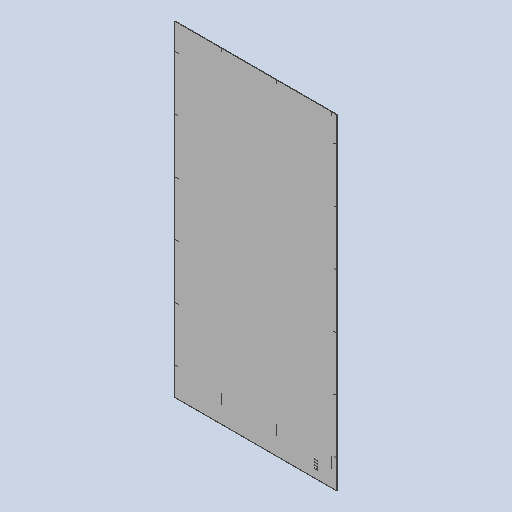
# Autodesk Inventor part: GBK 2221 shield 5
Saved by Autodesk Inventor 2026 (Build 300175000, 175)
## iProperties
Created: 2026-04-17
Part Number: GBK 2221 shield 5
Material: Steel
Document SubType Name: Sheet Metal
Designer: pokla
Stock Number: 2225
Mass: 138487 g
Surface Area: 88564.8 cm^2
Volume: 17641.6 cm^3
Density: 7.85 g/cm^3
Flat Pattern Width: 148 cm
Flat Pattern Length: 298 cm
Flat Pattern Area: 44104 cm^2
Sheet Metal Rule: По умолчанию_мм
Sheet Metal Width: 1480,000 мм
Sheet Metal Length: 2980,000 мм
Sheet Metal Area: 4410400,000 мм^2
Appearance: Default
Author: admin
Autodesk Inventor part; units mm, degrees
ref_plane "YZ Plane" through (0, 0, 0) normal (1, 0, 0) x (0, 1, 0)
ref_plane "XZ Plane" through (0, 0, 0) normal (0, 1, 0) x (-1, 0, 0)
ref_plane "XY Plane" through (0, 0, 0) normal (0, 0, 1) x (1, 0, 0)
sketch "Sketch1" plane through (0, 0, 0) normal (0, 0, 1) x (1, 0, 0)
  line L0 (740, -1490) -> (-740, -1490)
  line L1 (-740, -1490) -> (-740, 1490)
  line L2 (-740, 1490) -> (740, 1490)
  line L3 (740, 1490) -> (740, -1490)
  line L4 (740, -1490) -> (-740, 1490) construction
  line L5 (-740, -1490) -> (740, 1490) construction
  point P0 (0, 0)
  dimension "d0" = 1480
  dimension "d1" = 2980
  measures "d0" distance of L1.end L2.end
  measures "d1" distance of L0.end L1.end
extrude "Plate1" add sketch "Sketch1" along normal blind 4
sketch "Эскиз2" plane through (0, 0, 4) normal (0, 0, 1) x (1, 0, 0)
  line L0 (567.512, -1329.859) -> (567.512, -1827.9951) construction
  line L1 (567.512, -1827.9951) -> (527.8847, -1827.9951) construction
  line L2 (527.8847, -1827.9951) -> (527.8847, -1329.859) construction
  line L3 (527.8847, -1329.859) -> (567.512, -1329.859) construction
  line L4 (690.2486, -1238) -> (690.2486, -1335) projected
  line L5 (690.2486, -1335) -> (686.2496, -1335) projected
  line L6 (770, 1252.8333) -> (710, 1252.8333) projected
  line L7 (710, 1248.8333) -> (710, 1252.8333) projected
  line L8 (770, 756.1667) -> (710, 756.1667) projected
  line L9 (710, 752.1667) -> (710, 756.1667) projected
  line L10 (770, 259.5) -> (710, 259.5) projected
  line L11 (710, 255.5) -> (710, 259.5) projected
  line L12 (770, -237.1667) -> (710, -237.1667) projected
  line L13 (710, -241.1667) -> (710, -237.1667) projected
  line L14 (770, -733.8333) -> (710, -733.8333) projected
  line L15 (710, -737.8333) -> (710, -733.8333) projected
  line L16 (770, -1230.5) -> (710, -1230.5) projected
  line L17 (710, -1234.5) -> (710, -1230.5) projected
  line L18 (190.12, -1238) -> (190.12, -1335) projected
  line L19 (190.12, -1335) -> (186.121, -1335) projected
  line L20 (-310.0086, -1238) -> (-310.0086, -1335) projected
  line L21 (-310.0086, -1335) -> (-314.0076, -1335) projected
  ellipse E0 centre (690.2486, 1490.5) end of major axis (690.2486, 1520.5) minor radius 0.6803 (690.2486, 1460.5) -> (690.2486, 1520.5) ccw projected
  line L22 (690.2486, 1460.5) -> (686.2496, 1460.5) projected
  ellipse E1 centre (190.12, 1490.5) end of major axis (190.12, 1520.5) minor radius 0.6803 (190.12, 1460.5) -> (190.12, 1520.5) ccw projected
  line L23 (190.12, 1460.5) -> (186.121, 1460.5) projected
  ellipse E2 centre (-310.0086, 1490.5) end of major axis (-310.0086, 1520.5) minor radius 0.6803 (-310.0086, 1460.5) -> (-310.0086, 1520.5) ccw projected
  line L24 (-310.0086, 1460.5) -> (-314.0076, 1460.5) projected
  line L25 (-710, 1252.8333) -> (-739.3197, 1252.8333) projected
  line L26 (-710, 1248.8333) -> (-710, 1252.8333) projected
  line L27 (-710, 756.1667) -> (-739.3197, 756.1667) projected
  line L28 (-710, 752.1667) -> (-710, 756.1667) projected
  line L29 (-710, 259.5) -> (-739.3197, 259.5) projected
  line L30 (-710, 255.5) -> (-710, 259.5) projected
  line L31 (-710, -237.1667) -> (-739.3197, -237.1667) projected
  line L32 (-710, -241.1667) -> (-710, -237.1667) projected
  line L33 (-710, -733.8333) -> (-739.3197, -733.8333) projected
  line L34 (-710, -737.8333) -> (-710, -733.8333) projected
  line L35 (-710, -1230.5) -> (-739.3197, -1230.5) projected
  line L36 (-710, -1234.5) -> (-710, -1230.5) projected
  point P0 (0, 0)
  constraints: 5 other
mark "Маркировка1"
equation "\"d0\" = Лист_ширина"
equation "\"d2\" = Thickness"
equation "\"BendRadius\" = Thickness"
equation "\"BendReliefWidth\" = Thickness"
equation "\"BendReliefDepth\" = 0.5 * Thickness"
equation "\"CornerReliefSize\" = 4 * Thickness"
equation "\"MinimumRemnant\" = 2 * Thickness"
equation "\"TransitionRadius\" = BendRadius"
equation "\"JacobiRadiusSize\" = BendRadius"
equation "\"GapSize\" = Thickness"
equation "\"Лист_ширина\" = 1480"
equation "\"Thickness\" = 4"
body "Solid1"
